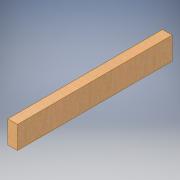
# Autodesk Inventor part: Top Continuation Bar
Saved by Autodesk Inventor 2018 (Build 220112000, 112)
## iProperties
Created: 2017-09-10
Part Number: Top Continuation Bar
Material: Wood
Document SubType Name: Modeling
Designer: jjsch
Density: 0.570257 g/cm^3
Appearance: Yellow Pine - Solid Natural Low Gloss
Mass: 1177.45 g
Surface Area: 1616.13 cm^2
Volume: 2064.77 cm^3
Author: jjsch
Autodesk Inventor part; units mm, degrees
ref_plane "YZ Plane" through (0, 0, 0) normal (1, 0, 0) x (0, 1, 0)
ref_plane "XZ Plane" through (0, 0, 0) normal (0, 1, 0) x (-1, 0, 0)
ref_plane "XY Plane" through (0, 0, 0) normal (0, 0, 1) x (1, 0, 0)
sketch "Sketch1" plane through (0, 0, 0) normal (1, 0, 0) x (0, 1, 0)
  line L0 (0, 0) -> (88.9, 0)
  line L1 (88.9, 0) -> (88.9, 609.6)
  line L2 (88.9, 609.6) -> (0, 609.6)
  line L3 (0, 609.6) -> (0, 0)
  dimension "d0" = 88.9
  dimension "d1" = 609.6
  constraints: 8 end point, 2 parallel, 1 horizontal, 1 perpendicular
  measures "d0" distance of L2.end L1.end
  measures "d1" distance of L1.end L0.end
extrude "Extrusion1" add sketch "Sketch1" along normal blind 38.1
body "Solid1"
